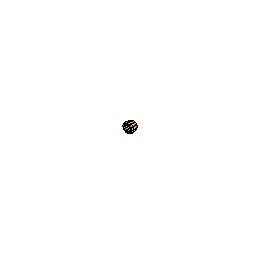
Collet (Autodesk Fusion 360 design; units mm, degrees)
Autodesk Fusion 360 part; units mm, degrees
note: some values were not read from the file. Set by a fixed rule: which sketch regions a step uses.
sketch "Sketch4" plane through (0, 0, 0) normal (0, 0, 1) x (1, 0, 0)
  line L0 (-8.2935, 11) -> (8.2935, 11)
  line L1 (12.9007, 11) -> (1.0917, 11)
  line L2 (1.0917, 11) -> (-1.0917, 11)
  line L3 (-1.0917, 11) -> (-12.9007, 11)
  line L4 (10.4508, 11) -> (-10.4508, 11)
  line L5 (7.2537, -4) -> (-7.2537, -4)
  line L6 (12.1, -4) -> (5.012, -4)
  line L7 (5.012, -4) -> (-5.012, -4)
  line L8 (-5.012, -4) -> (-12.1, -4)
  line L9 (-12.1, -4) -> (-5.012, -4)
  line L10 (-5.012, -4) -> (5.012, -4)
  line L11 (5.012, -4) -> (12.1, -4)
  line L12 (8.8, 11) -> (5.1988, -4)
  line L13 (6.9399, 11) -> (6.9399, -4)
  line L14 (8.8, 11) -> (8.2935, -4)
  line L15 (5.1988, -4) -> (8.2935, -4)
  line L16 (7.2537, 0) -> (-7.2537, 0)
  line L17 (-8.2935, 11) -> (8.2935, 11)
  line L18 (8.8, 11) -> (7.2537, 0)
  point P0 (0, 11)
  dimension "d1" = 103.5
  dimension "d2" = 8.8
  constraint coincident L1 L12.start
  constraint coincident L6 L12.end
  constraint coincident L0 L13.start
  constraint coincident L11 L13.end
  constraint perpendicular L0 L13
  constraint midpoint L0 P0
  constraint coincident L6 L14.end
  constraint parallel L11 L15
  constraint coincident L16.start L18.end
  measures "d1" angle of L1 L12
  measures "d2" distance of L12.start P0
sketch "Sketch1" plane through (0, 0, 0) normal (0, 0, 1) x (1, 0, 0)
  line L0 (0, 0) -> (6, 0) construction
  line L1 (6, 0) -> (7.67, 0)
  line L2 (7.67, 0) -> (9, 3)
  line L3 (9, 3) -> (6.835, 12)
  line L4 (6.835, 12) -> (6, 12)
  line L5 (6, 12) -> (6, 0)
  dimension "d15" = 6
  dimension "d16" = 1.67
  dimension "d17" = 0.835
  dimension "d18" = 3
  dimension "d19" = 3
  dimension "d20" = 12
  dimension "d97" = 113.909
  dimension "d117" = 103.526
  constraint coincident L0.start origin
  constraint horizontal L0
  constraint parallel L0 L1
  constraint parallel L0 L4
  constraint perpendicular L1 L5
  measures "d15" distance of L0.start L0.end
  measures "d16" distance of L0.end L1.end
  measures "d17" distance of L3.end L4.end
  measures "d18" distance of L2.end L5
  measures "d19" vertical distance of L1.end L2.end
  measures "d20" distance of L0.end L4.end
  measures "d97" angle of L1 L2
  measures "d117" angle of L3 L4
revolve "Revolve1" add sketch "Sketch1" angle 360 about axis through (0, -205.75, 0) along (0, 1, 0)
sketch "Sketch2" plane through (0, 0, 0) normal (0, -1, 0) x (1, 0, 0)
  circle A0 centre (0, 0) radius 7.67
  circle A1 centre (0, 0) radius 6
  circle A2 centre (0, 0) radius 9 construction
  line L0 (-9, 0) -> (9, 0) construction
  line L1 (4.5, 7.7942) -> (-4.5, -7.7942) construction
  line L2 (-4.5, 7.7942) -> (4.5, -7.7942) construction
  line L3 (-4.933, 7.5442) -> (-4.067, 8.0442)
  line L4 (-4.067, 8.0442) -> (4.933, -7.5442)
  line L5 (4.933, -7.5442) -> (4.067, -8.0442)
  line L6 (4.067, -8.0442) -> (-4.933, 7.5442)
  line L7 (4.067, 8.0442) -> (4.933, 7.5442)
  line L8 (4.933, 7.5442) -> (-4.067, -8.0442)
  line L9 (-4.067, -8.0442) -> (-4.933, -7.5442)
  line L10 (-4.933, -7.5442) -> (4.067, 8.0442)
  line L11 (-9, 0.5) -> (9, 0.5)
  line L12 (9, 0.5) -> (9, -0.5)
  line L13 (9, -0.5) -> (-9, -0.5)
  line L14 (-9, -0.5) -> (-9, 0.5)
  dimension "d22" = 60
  dimension "d23" = 60
  dimension "d25" = 1
  dimension "d26" = 1
  dimension "d27" = 1
  constraint horizontal L0
  constraint coincident A0.centre L2
  constraint coincident A0.centre L0
  constraint coincident A0.centre L1
  constraint coincident A2 L0.start
  constraint coincident A2 L1.end
  constraint coincident A2 L2.start
  constraint coincident A2 L1.start
  constraint coincident A2 L2.end
  constraint coincident A2 L0.end
  constraint perpendicular L2 L3
  constraint perpendicular L3 L4
  constraint perpendicular L4 L5
  constraint perpendicular L8 L9
  constraint horizontal L11
  constraint perpendicular L11 L12
  constraint parallel L1 L10
  constraint parallel L1 L8
  constraint parallel L0 L13
  constraint perpendicular L13 L14
  constraint perpendicular L7 L10
  constraint midpoint L2.start L3
  constraint midpoint L2.end L5
  constraint midpoint L1.end L9
  constraint midpoint L1.start L7
  constraint midpoint L0.start L14
  constraint midpoint L0.end L12
  measures "d22" angle of L0 L1
  measures "d23" angle of L0 L2
  measures "d25" distance of L7.start L7.end
  measures "d26" distance of L3.start L3.end
  measures "d27" distance of L11.end L12.end
extrude "Extrude1" cut sketch "Sketch2" against normal blind 11 contours A0 A1 L11 L13 | A0 L11 L12 L13 | A0 A1 L8 L10 | A0 L7 L8 L10 | A0 L4 L5 L6 | A0 A1 L4 L6 | A0 A1 L4 L6 | A0 L3 L4 L6 | A0 L8 L9 L10 | A0 A1 L8 L10 | A0 A1 L11 L13 | A0 L11 L13 L14
fillet "Fillet1" radius 0.5 12 edges at (-2.8262, 11, 5.8952) (-3.6923, 11, 5.3952) (2.8262, 11, 5.8952) (3.6923, 11, 5.3952) (6.5185, 11, 0.5) (6.5185, 11, -0.5) (3.6923, 11, -5.3952) (2.8262, 11, -5.8952) (-2.8262, 11, -5.8952) (-3.6923, 11, -5.3952) (-6.5185, 11, -0.5) (-6.5185, 11, 0.5)
sketch "Sketch3" plane through (0, 12, 0) normal (0, 1, 0) x (-1, 0, 0)
  line L0 (0.5, -9) -> (-0.5, -9)
  line L1 (-0.5, -9) -> (-0.5, 9)
  line L2 (-0.5, 9) -> (0.5, 9)
  line L3 (0.5, 9) -> (0.5, -9)
  line L4 (7.5442, -4.933) -> (-8.0442, 4.067)
  line L5 (-8.0442, 4.067) -> (-7.5442, 4.933)
  line L6 (-7.5442, 4.933) -> (8.0442, -4.067)
  line L7 (8.0442, -4.067) -> (7.5442, -4.933)
  line L8 (-7.5442, -4.933) -> (8.0442, 4.067)
  line L9 (8.0442, 4.067) -> (7.5442, 4.933)
  line L10 (7.5442, 4.933) -> (-8.0442, -4.067)
  line L11 (-8.0442, -4.067) -> (-7.5442, -4.933)
  line L12 (0, -9) -> (0, 9) construction
  line L13 (7.7942, 4.5) -> (-7.7942, -4.5) construction
  line L14 (7.7942, -4.5) -> (-7.7942, 4.5) construction
  arc A0 (8.9861, 0.5) -> (4.9261, 7.5322) centre (0, 0) ccw construction
  arc A1 (4.06, 8.0322) -> (-4.06, 8.0322) centre (0, 0) ccw construction
  arc A2 (-4.9261, 7.5322) -> (-8.9861, 0.5) centre (0, 0) ccw construction
  arc A3 (-8.9861, -0.5) -> (-4.9261, -7.5322) centre (0, 0) ccw construction
  arc A4 (-4.06, -8.0322) -> (4.06, -8.0322) centre (0, 0) ccw construction
  arc A5 (4.9261, -7.5322) -> (8.9861, -0.5) centre (0, 0) ccw construction
  circle A6 centre (0, 0) radius 6
  circle A7 centre (0, 0) radius 6.835
  dimension "d98" = 60
  dimension "d99" = 60
  dimension "d100" = 1
  dimension "d101" = 1
  dimension "d102" = 1
  constraint horizontal L0
  constraint perpendicular L0 L1
  constraint perpendicular L1 L2
  constraint perpendicular L4 L5
  constraint perpendicular L8 L9
  constraint perpendicular L9 L10
  constraint perpendicular L8 L11
  constraint perpendicular L4 L7
  constraint perpendicular L6 L7
  constraint perpendicular L2 L3
  constraint midpoint L0 L12.start
  constraint midpoint L2 L12.end
  constraint midpoint L9 L13.start
  constraint midpoint L11 L13.end
  constraint perpendicular L11 L13
  constraint midpoint L7 L14.start
  constraint midpoint L5 L14.end
  constraint perpendicular L5 L14
  constraint coincident A0.centre L14
  constraint coincident A0.centre L13
  constraint coincident A0.centre L12
  constraint coincident L13.start A0
  constraint coincident L12.end A1
  constraint coincident L14.end A2
  constraint coincident L13.end A3
  constraint coincident L12.start A4
  constraint coincident L14.start A5
  measures "d98" angle of L12 L13
  measures "d99" angle of L13 L14
  measures "d100" distance of L0.start L0.end
  measures "d101" distance of L8.start L10.end
  measures "d102" distance of L4.end L5.end
extrude "Extrude2" cut sketch "Sketch3" against normal blind 11 contours L0 L1 L3 A7 | L1 L3 A6 A7 | L4 L6 L7 A7 | L4 L6 A6 A7 | L8 L10 A6 A7 | L8 L10 L11 A7 | L4 L6 A6 A7 | L4 L5 L6 A7 | L8 L9 L10 A7 | L8 L10 A6 A7 | L1 L3 A6 A7 | L1 L2 L3 A7
fillet "Fillet2" radius 0.5 12 edges at (-0.5, 1, 7.0385) (0.5, 1, 7.0385) (-5.8455, 1, 3.9523) (-6.3455, 1, 3.0862) (-6.3455, 1, -3.0862) (-5.8455, 1, -3.9523) (-0.5, 1, -7.0385) (0.5, 1, -7.0385) (6.3455, 1, -3.0862) (5.8455, 1, -3.9523) (6.3455, 1, 3.0862) (5.8455, 1, 3.9523)
revolve "Revolve2" [suppressed]
equation "d17 = 1.67 mm / 2"
equation "d25 = d27"
equation "d26 = d27"
equation "d101 = d100"
equation "d102 = d100"
named bodies: "Collet"
